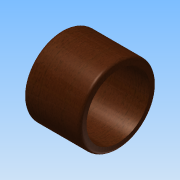
# Autodesk Inventor part: RubberGrip
Saved by Autodesk Inventor 2015 (Build 190159000, 159)
## iProperties
Created: 2016-11-08
Part Number: RubberGrip
Material: Wood (Walnut)
Document SubType Name: Modeling
Designer: Aniket Pant
Density: 0.55 g/cm^3
Appearance: Walnut - Natural Polished
Author: Aniket Pant
Autodesk Inventor part; units mm, degrees
ref_plane "YZ Plane" through (0, 0, 0) normal (1, 0, 0) x (0, 1, 0)
ref_plane "XZ Plane" through (0, 0, 0) normal (0, 1, 0) x (-1, 0, 0)
ref_plane "XY Plane" through (0, 0, 0) normal (0, 0, 1) x (1, 0, 0)
sketch "Sketch1" plane through (0, 0, 0) normal (0, 0, 1) x (1, 0, 0)
  line L0 (0, 0) -> (3.9624, 0)
  line L1 (3.9624, 0) -> (3.9624, -46.3015)
  line L2 (16.4707, -59.9969) -> (0, -59.9969)
  line L3 (0, -59.9969) -> (0, 0)
  line L4 (0, -59.9969) -> (113.5126, -59.9969)
  line L5 (113.5126, -59.9969) -> (113.5126, -46.3015)
  line L6 (113.5126, -46.3015) -> (3.9624, -46.3015)
  line L7 (0, -46.3015) -> (0, -59.9969)
  line L8 (-58.687, 17.3919) -> (148.6234, 17.3919) construction
  dimension "d0" = 113.5126
  dimension "d1" = 3.9624
  dimension "d2" = 13.6954
  dimension "d3" = 46.3015
  constraints: 18 end point, 4 parallel, 3 horizontal, 2 perpendicular
  measures "d0" distance of L2.end L4.end
  measures "d1" distance of L0.start L0.end
  measures "d2" distance of L4.end L5.end
  measures "d3" distance of L0.end L1.end
revolve "Revolution1" add sketch "Sketch1" angle 360 about axis through (-58.687, 17.3919, 0) along (1, 0, 0)
fillet "Fillet1" radius 6.35 2 edges at (113.5126, 94.7807, 0) (0, 94.7807, 0)
body "Solid1"
